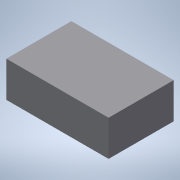
# Autodesk Inventor part: Carroserie 1.0
Saved by Autodesk Inventor 2021 (Build 250183000, 183)
## iProperties
Created: 2020-10-29
Part Number: Carroserie 1.0
Material: Generic
Document SubType Name: Modeling
Designer: buele
Density: 1 g/cm^3
Appearance: Default
Author: buele
Autodesk Inventor part; units mm, degrees
ref_plane "YZ Plane" through (0, 0, 0) normal (1, 0, 0) x (0, 1, 0)
ref_plane "XZ Plane" through (0, 0, 0) normal (0, 1, 0) x (-1, 0, 0)
ref_plane "XY Plane" through (0, 0, 0) normal (0, 0, 1) x (1, 0, 0)
sketch "Sketch1" plane through (0, 0, 0) normal (0, 0, 1) x (1, 0, 0)
  line L0 (-14.3723, 10.3315) -> (14.3286, 10.3315)
  line L1 (14.3286, 10.3315) -> (14.3286, -7.9288)
  line L2 (14.3286, -7.9288) -> (-14.3723, -7.9288)
  line L3 (-14.3723, -7.9288) -> (-14.3723, 10.3315)
  point P0 (0, 0)
  constraints: 8 end point, 2 parallel, 1 horizontal, 1 perpendicular
extrude "Extrusion1" add sketch "Sketch1" along normal blind 10
body "Solid1"
